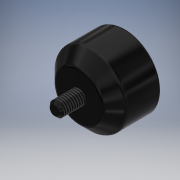
# Autodesk Inventor part: Motor
Saved by Autodesk Inventor 2019 (Build 230136000, 136)
## iProperties
Created: 2019-10-06
Part Number: Motor
Material: UHMW, Black
Document SubType Name: Modeling
Designer: robgr
Density: 0.94 g/cm^3
Appearance: Smooth - Black
Mass: 21.6282 g
Surface Area: 55.0499 cm^2
Volume: 23.0087 cm^3
Author: robgr
Autodesk Inventor part; units mm, degrees
ref_plane "XY Plane" through (0, 0, 0) normal (0, 0, 1) x (1, 0, 0)
sketch "Sketch1" plane through (0, 0, 0) normal (0, 0, 1) x (1, 0, 0)
  circle A0 centre (0, 0) radius 15
  dimension "d0" = 30
  constraints: 1 centre point, 1 coincident
  measures "d0" diameter of A0
extrude "Extrusion1" add sketch "Sketch1" along normal blind 20
sketch "Sketch3" plane through (0, 0, 20) normal (0, 0, 1) x (1, 0, 0)
  circle A0 centre (0, 0) radius 15
  constraints: 1 centre point, 1 coincident
extrude "Extrusion3" add sketch "Sketch3" along normal blind 1
chamfer "Chamfer1" distance 5 angle 45 1 edges at (-15, 0, 21)
fillet "Fillet1" radius 2 2 edges at (-15, 0, 16) (-10, 0, 21)
sketch "Sketch4" plane through (0, 0, 21) normal (0, 0, 1) x (1, 0, 0)
  circle A0 centre (0, 0) radius 3
  dimension "d12" = 6
  constraints: 1 centre point, 1 coincident
  measures "d12" diameter of A0
extrude "Extrusion4" add sketch "Sketch4" along normal blind 10
chamfer "Chamfer2" distance 1 angle 45 1 edges at (-3, 0, 31)
fillet "Fillet2" radius 1 1 edges at (-15, 0, 0)
ref_plane "Work Plane2" through (0, 14.5, 0) normal (0, 1, 0) x (-1, 0, 0)
ref_plane "Work Plane1" through (0, -15.5, 0) normal (0, 1, 0) x (-1, 0, 0)
ref_plane "Work Plane3" through (-14.75, 0, 0) normal (1, 0, 0) x (0, 1, 0)
sketch "Sketch5" plane through (-14.75, 0, 0) normal (1, 0, 0) x (0, 1, 0)
  line L0 (7.5, 2.5) -> (-7.5, 2.5)
  line L1 (-7.5, 2.5) -> (-7.5, 14.5)
  line L2 (-7.5, 14.5) -> (7.5, 14.5)
  line L3 (7.5, 14.5) -> (7.5, 2.5)
  line L4 (9.8328, 18.3373) -> (9.8328, 18.1192)
  line L5 (7.5, 12.0972) -> (7.5, 12.3154)
  line L6 (-15, 1) -> (15, 1) projected
  line L7 (15, 1) -> (15, 15.1716) projected
  line L8 (-15, 1) -> (15, 1)
  line L9 (15, 1) -> (15, 15.1716)
  line L10 (15, 15.1716) -> (-15, 15.1716)
  line L11 (-15, 15.1716) -> (-15, 1)
  line L12 (15, 15.1716) -> (-15, 15.1716) projected
  point P0 (0, 0)
  dimension "d28" = 15
  dimension "d29" = 12
  dimension "d30" = 7.5
  dimension "d31" = 7.5
  dimension "d32" = 1.5
  dimension "d34" = 0
  constraints: 20 end point, 5 parallel, 2 horizontal, 2 perpendicular, 2 point on line
  measures "d28" distance of L1.end L2.end
  measures "d29" distance of L2.end L0.start
  measures "d30" distance between parallel lines of L11 L1
  measures "d31" distance between parallel lines of L7 L3
  measures "d32" distance between parallel lines of L6 L0
  measures "d34" distance between parallel lines of L10 L12
extrude "Extrusion5" cut sketch "Sketch5" along normal blind 20 and the other way blind 5 contours L0 L1 L2 L3
thread "Thread1" size "M6x1" class "6g" standard "ANSI Metric M Profile" full length
sketch "Sketch6" plane through (5.25, 0, 0) normal (-1, 0, 0) x (0, 0, 1)
  line L0 (0, -16.1407) -> (1.4634, -16.1407)
  line L1 (1.4634, -16.1407) -> (1.4634, 17.2598)
  line L2 (1.4634, 17.2598) -> (0, 17.2598)
  line L3 (0, 17.2598) -> (0, -16.1407)
  point P0 (0, 0)
  constraints: 8 end point, 2 parallel, 1 horizontal, 1 perpendicular
extrude "Extrusion6" cut sketch "Sketch6" along normal through all both and the other way through all
fillet "Fillet3" radius 1 1 edges at (-15, 0, 1.4634)
body "Solid1"
